Autodesk Fusion 360 part; units mm, degrees
note: some values were not read from the file. Set by a fixed rule: which sketch regions a step uses.
(part 12 of 15)
  line L9703 (42.4168, -64.2747) -> (42.4728, -64.098)
  line L9704 (145.736, -64.6246) -> (145.454, -64.6312)
  line L9705 (143.987, -63.884) -> (143.827, -63.6515)
  line L9706 (184.335, -62.7681) -> (184.478, -62.8863)
  line L9707 (145.579, -60.6337) -> (145.861, -60.6581)
  line L9708 (147.166, -63.809) -> (146.984, -64.0253)
  line L9709 (147.544, -62.759) -> (147.506, -63.039)
  line L9710 (147.43, -63.3109) -> (147.316, -63.5693)
  line L9711 (146.015, -64.5782) -> (145.736, -64.6246)
  line L9712 (145.173, -64.598) -> (144.9, -64.5256)
  line L9713 (147.528, -62.3517) -> (147.548, -62.6335)
  line L9714 (146.4, -60.8238) -> (146.646, -60.9619)
  line L9715 (184.753, -63.5822) -> (184.73, -63.7661)
  line L9716 (143.752, -61.7536) -> (143.894, -61.5093)
  line L9717 (188.432, -64.6381) -> (188.159, -64.5657)
  line L9718 (143.578, -62.2896) -> (143.646, -62.0154)
  line L9719 (144.503, -60.9282) -> (144.754, -60.798)
  line L9720 (144.273, -61.0924) -> (144.503, -60.9282)
  line L9721 (184.172, -62.6799) -> (184.335, -62.7681)
  line L9722 (184.478, -62.8863) -> (184.595, -63.0299)
  line L9723 (145.02, -60.7044) -> (145.297, -60.6492)
  line L9724 (144.069, -61.2874) -> (144.273, -61.0924)
  line L9725 (146.984, -64.0253) -> (146.774, -64.2138)
  line L9726 (189.543, -64.5331) -> (189.273, -64.6183)
  line L9727 (145.861, -60.6581) -> (146.136, -60.7219)
  line L9728 (190.807, -62.6735) -> (190.803, -62.7991)
  line L9729 (188.279, -60.7444) -> (188.556, -60.6893)
  line L9730 (184.595, -63.0299) -> (184.682, -63.1936)
  line L9731 (144.9, -64.5256) -> (144.64, -64.4155)
  line L9732 (147.069, -61.3346) -> (147.237, -61.5618)
  line L9733 (146.646, -60.9619) -> (146.871, -61.1332)
  line L9734 (146.871, -61.1332) -> (147.069, -61.3346)
  line L9735 (187.01, -61.7937) -> (187.152, -61.5494)
  line L9736 (184.682, -63.1936) -> (184.736, -63.3711)
  line L9737 (184.73, -63.7661) -> (184.672, -63.9421)
  line L9738 (186.904, -62.0555) -> (187.01, -61.7937)
  line L9739 (184.672, -63.9421) -> (184.58, -64.1033)
  line L9740 (147.371, -61.8104) -> (147.469, -62.0755)
  line L9741 (187.532, -61.1325) -> (187.762, -60.9683)
  line L9742 (188.159, -64.5657) -> (187.899, -64.4555)
  line L9743 (147.506, -63.039) -> (147.43, -63.3109)
  line L9744 (147.237, -61.5618) -> (147.371, -61.8104)
  line L9745 (147.316, -63.5693) -> (147.166, -63.809)
  line L9746 (146.539, -64.3707) -> (146.284, -64.493)
  line L9747 (190.032, -64.2538) -> (189.797, -64.4108)
  line L9748 (190.495, -61.6019) -> (190.629, -61.8505)
  line L9749 (188.012, -60.838) -> (188.279, -60.7444)
  line L9750 (187.327, -61.3275) -> (187.532, -61.1325)
  line L9751 (189.273, -64.6183) -> (188.995, -64.6647)
  line L9752 (188.556, -60.6893) -> (188.838, -60.6738)
  line L9753 (146.136, -60.7219) -> (146.4, -60.8238)
  line L9754 (188.838, -60.6738) -> (189.119, -60.6982)
  line L9755 (146.284, -64.493) -> (146.015, -64.5782)
  line L9756 (147.548, -62.6335) -> (147.544, -62.759)
  line L9757 (145.454, -64.6312) -> (145.173, -64.598)
  line L9758 (183.995, -62.6251) -> (184.172, -62.6799)
  line L9759 (143.549, -62.5706) -> (143.578, -62.2896)
  line L9760 (144.754, -60.798) -> (145.02, -60.7044)
  line L9761 (143.646, -62.0154) -> (143.752, -61.7536)
  line L9762 (187.762, -60.9683) -> (188.012, -60.838)
  line L9763 (147.469, -62.0755) -> (147.528, -62.3517)
  line L9764 (189.797, -64.4108) -> (189.543, -64.5331)
  line L9765 (145.297, -60.6492) -> (145.579, -60.6337)
  line L9766 (187.152, -61.5494) -> (187.327, -61.3275)
  line L9767 (146.774, -64.2138) -> (146.539, -64.3707)
  line L9768 (182.869, -63.7272) -> (182.854, -63.5424)
  line L9769 (306.287, -60.7875) -> (306.455, -61.0148)
  line L9770 (182.874, -63.3581) -> (182.931, -63.1814)
  line L9771 (151.5, -63.5421) -> (151.477, -63.7261)
  line L9772 (151.342, -62.9899) -> (151.429, -63.1536)
  line L9773 (183.262, -64.3358) -> (183.12, -64.2156)
  line L9774 (182.92, -63.9054) -> (182.869, -63.7272)
  line L9775 (150.373, -62.5824) -> (150.557, -62.5656)
  line L9776 (151.327, -64.0632) -> (151.206, -64.2036)
  line L9777 (149.678, -63.1414) -> (149.767, -62.9789)
  line L9778 (183.81, -62.6057) -> (183.995, -62.6251)
  line L9779 (151.429, -63.1536) -> (151.483, -63.3311)
  line L9780 (150.195, -62.6348) -> (150.373, -62.5824)
  line L9781 (149.767, -62.9789) -> (149.886, -62.8368)
  line L9782 (183.969, -64.4912) -> (183.784, -64.5055)
  line L9783 (149.616, -63.6871) -> (149.601, -63.5023)
  line L9784 (183.448, -62.6748) -> (183.626, -62.6225)
  line L9785 (184.736, -63.3711) -> (184.754, -63.5557)
  line L9786 (184.754, -63.5557) -> (184.753, -63.5822)
  line L9787 (144.179, -64.0914) -> (143.987, -63.884)
  line L9788 (183.02, -63.0189) -> (183.139, -62.8769)
  line L9789 (150.919, -62.6398) -> (151.082, -62.728)
  line L9790 (151.419, -63.902) -> (151.327, -64.0632)
  line L9791 (305.079, -60.111) -> (305.354, -60.1748)
  line L9792 (184.313, -64.3578) -> (184.147, -64.4414)
  line L9793 (150.009, -64.2957) -> (149.867, -64.1755)
  line L9794 (149.886, -62.8368) -> (150.031, -62.7207)
  line L9795 (150.17, -64.3861) -> (150.009, -64.2957)
  line L9796 (151.483, -63.3311) -> (151.501, -63.5156)
  line L9797 (183.423, -64.4262) -> (183.262, -64.3358)
  line L9798 (143.56, -62.8529) -> (143.549, -62.5706)
  line L9799 (143.894, -61.5093) -> (144.069, -61.2874)
  line L9800 (183.284, -62.7607) -> (183.448, -62.6748)
  line L9801 (184.147, -64.4414) -> (183.969, -64.4912)
  line L9802 (184.58, -64.1033) -> (184.459, -64.2436)
  line L9803 (306.687, -61.5284) -> (306.746, -61.8046)
  line L9804 (143.7, -63.3988) -> (143.611, -63.1308)
  line L9805 (149.752, -64.0302) -> (149.668, -63.8653)
  line L9806 (306.589, -61.2634) -> (306.687, -61.5284)
  line L9807 (183.626, -62.6225) -> (183.81, -62.6057)
  line L9808 (151.206, -64.2036) -> (151.06, -64.3177)
  line L9809 (149.668, -63.8653) -> (149.616, -63.6871)
  line L9810 (144.398, -64.2698) -> (144.179, -64.0914)
  line L9811 (143.827, -63.6515) -> (143.7, -63.3988)
  line L9812 (183.6, -64.4835) -> (183.423, -64.4262)
  line L9813 (151.225, -62.8462) -> (151.342, -62.9899)
  line L9814 (151.501, -63.5156) -> (151.5, -63.5421)
  line L9815 (182.854, -63.5424) -> (182.874, -63.3581)
  line L9816 (183.139, -62.8769) -> (183.284, -62.7607)
  line L9817 (182.931, -63.1814) -> (183.02, -63.0189)
  line L9818 (183.784, -64.5055) -> (183.6, -64.4835)
  line L9819 (149.622, -63.3181) -> (149.678, -63.1414)
  line L9820 (305.618, -60.2768) -> (305.864, -60.4148)
  line L9821 (150.031, -62.7207) -> (150.195, -62.6348)
  line L9822 (151.082, -62.728) -> (151.225, -62.8462)
  line L9823 (151.06, -64.3177) -> (150.894, -64.4013)
  line L9824 (151.477, -63.7261) -> (151.419, -63.902)
  line L9825 (183.12, -64.2156) -> (183.005, -64.0703)
  line L9826 (150.716, -64.4512) -> (150.531, -64.4654)
  line L9827 (150.742, -62.585) -> (150.919, -62.6398)
  line L9828 (144.64, -64.4155) -> (144.398, -64.2698)
  line L9829 (143.611, -63.1308) -> (143.56, -62.8529)
  line L9830 (184.459, -64.2436) -> (184.313, -64.3578)
  line L9831 (183.005, -64.0703) -> (182.92, -63.9054)
  line L9832 (306.202, -63.4782) -> (305.992, -63.6667)
  line L9833 (303.858, -63.8684) -> (303.616, -63.7227)
  line L9834 (302.864, -61.4684) -> (302.97, -61.2065)
  line L9835 (306.384, -63.262) -> (306.202, -63.4782)
  line L9836 (305.233, -64.0312) -> (304.954, -64.0775)
  line L9837 (302.97, -61.2065) -> (303.112, -60.9622)
  line L9838 (306.089, -60.5862) -> (306.287, -60.7875)
  line L9839 (302.767, -62.0236) -> (302.796, -61.7426)
  line L9840 (303.491, -60.5454) -> (303.721, -60.3811)
  line L9841 (303.287, -60.7404) -> (303.491, -60.5454)
  line L9842 (303.397, -63.5444) -> (303.205, -63.3369)
  line L9843 (306.766, -62.0864) -> (306.762, -62.212)
  line L9844 (31.5843, -62.1719) -> (31.5467, -62.4519)
  line L9845 (30.6863, -60.3747) -> (30.9109, -60.5461)
  line L9846 (306.648, -62.7639) -> (306.534, -63.0223)
  line L9847 (303.972, -60.2509) -> (304.238, -60.1573)
  line L9848 (31.2769, -60.9747) -> (31.4111, -61.2233)
  line L9849 (302.829, -62.5838) -> (302.778, -62.3059)
  line L9850 (303.721, -60.3811) -> (303.972, -60.2509)
  line L9851 (304.672, -64.0842) -> (304.391, -64.051)
  line L9852 (31.1091, -60.7475) -> (31.2769, -60.9747)
  line L9853 (30.0552, -63.9911) -> (29.7765, -64.0375)
  line L9854 (29.494, -64.0441) -> (29.2135, -64.0109)
  line L9855 (28.4383, -63.6826) -> (28.2192, -63.5043)
  line L9856 (303.616, -63.7227) -> (303.397, -63.5444)
  line L9857 (305.354, -60.1748) -> (305.618, -60.2768)
  line L9858 (29.2135, -64.0109) -> (28.9404, -63.9385)
  line L9859 (30.1763, -60.1348) -> (30.4398, -60.2367)
  line L9860 (302.918, -62.8518) -> (302.829, -62.5838)
  line L9861 (30.8141, -63.6267) -> (30.5792, -63.7836)
  line L9862 (306.725, -62.492) -> (306.648, -62.7639)
  line L9863 (305.992, -63.6667) -> (305.757, -63.8237)
  line L9864 (303.205, -63.3369) -> (303.045, -63.1045)
  line L9865 (304.118, -63.9786) -> (303.858, -63.8684)
  line L9866 (30.5792, -63.7836) -> (30.3245, -63.9059)
  line L9867 (31.3558, -62.9822) -> (31.2063, -63.2219)
  line L9868 (305.502, -63.946) -> (305.233, -64.0312)
  line L9869 (28.6803, -63.8284) -> (28.4383, -63.6826)
  line L9870 (31.5467, -62.4519) -> (31.47, -62.7238)
  line L9871 (306.455, -61.0148) -> (306.589, -61.2634)
  line L9872 (302.796, -61.7426) -> (302.864, -61.4684)
  line L9873 (306.534, -63.0223) -> (306.384, -63.262)
  line L9874 (303.045, -63.1045) -> (302.918, -62.8518)
  line L9875 (303.112, -60.9622) -> (303.287, -60.7404)
  line L9876 (304.391, -64.051) -> (304.118, -63.9786)
  line L9877 (304.954, -64.0775) -> (304.672, -64.0842)
  line L9878 (306.762, -62.212) -> (306.725, -62.492)
  line L9879 (302.778, -62.3059) -> (302.767, -62.0236)
  line L9880 (305.757, -63.8237) -> (305.502, -63.946)
  line L9881 (29.7765, -64.0375) -> (29.494, -64.0441)
  line L9882 (31.5883, -62.0463) -> (31.5843, -62.1719)
  line L9883 (28.2192, -63.5043) -> (28.0274, -63.2968)
  line L9884 (28.9404, -63.9385) -> (28.6803, -63.8284)
  line L9885 (150.531, -64.4654) -> (150.347, -64.4434)
  line L9886 (306.746, -61.8046) -> (306.766, -62.0864)
  line L9887 (30.3245, -63.9059) -> (30.0552, -63.9911)
  line L9888 (304.516, -60.1022) -> (304.798, -60.0867)
  line L9889 (29.9011, -60.071) -> (30.1763, -60.1348)
  line L9890 (305.864, -60.4148) -> (306.089, -60.5862)
  line L9891 (149.867, -64.1755) -> (149.752, -64.0302)
  line L9892 (150.347, -64.4434) -> (150.17, -64.3861)
  line L9893 (150.894, -64.4013) -> (150.716, -64.4512)
  line L9894 (149.601, -63.5023) -> (149.622, -63.3181)
  line L9895 (150.557, -62.5656) -> (150.742, -62.585)
  line L9896 (35.2652, -62.2591) -> (35.3824, -62.4028)
  line L9897 (300.107, -63.8543) -> (299.928, -63.9041)
  line L9898 (299.221, -63.7486) -> (299.08, -63.6285)
  line L9899 (31.2063, -63.2219) -> (31.0245, -63.4382)
  line L9900 (300.713, -62.9685) -> (300.713, -62.9951)
  line L9901 (300.295, -62.181) -> (300.438, -62.2991)
  line L9902 (299.744, -63.9183) -> (299.559, -63.8964)
  line L9903 (35.5175, -63.139) -> (35.459, -63.3149)
  line L9904 (298.834, -62.771) -> (298.89, -62.5943)
  line L9905 (30.4398, -60.2367) -> (30.6863, -60.3747)
  line L9906 (31.5683, -61.7645) -> (31.5883, -62.0463)
  line L9907 (34.7821, -61.9979) -> (34.9592, -62.0527)
  line L9908 (35.3824, -62.4028) -> (35.4694, -62.5665)
  line L9909 (299.954, -62.038) -> (300.132, -62.0928)
  line L9910 (299.383, -63.8391) -> (299.221, -63.7486)
  line L9911 (35.459, -63.3149) -> (35.3674, -63.4761)
  line L9912 (27.6511, -62.5437) -> (27.6003, -62.2658)
  line L9913 (300.419, -63.6565) -> (300.272, -63.7707)
  line L9914 (27.7405, -62.8117) -> (27.6511, -62.5437)
  line L9915 (31.47, -62.7238) -> (31.3558, -62.9822)
  line L9916 (31.4111, -61.2233) -> (31.5088, -61.4884)
  line L9917 (28.794, -60.2108) -> (29.0605, -60.1172)
  line L9918 (27.7922, -61.1665) -> (27.9341, -60.9222)
  line L9919 (28.109, -60.7003) -> (28.3134, -60.5053)
  line L9920 (304.798, -60.0867) -> (305.079, -60.111)
  line L9921 (300.642, -62.6065) -> (300.695, -62.784)
  line L9922 (28.0274, -63.2968) -> (27.8668, -63.0644)
  line L9923 (300.631, -63.3549) -> (300.54, -63.5162)
  line L9924 (300.555, -62.4428) -> (300.642, -62.6065)
  line L9925 (300.272, -63.7707) -> (300.107, -63.8543)
  line L9926 (28.5433, -60.3411) -> (28.794, -60.2108)
  line L9927 (31.0245, -63.4382) -> (30.8141, -63.6267)
  line L9928 (27.618, -61.7025) -> (27.6861, -61.4283)
  line L9929 (298.98, -62.4318) -> (299.099, -62.2898)
  line L9930 (29.3376, -60.0621) -> (29.6197, -60.0466)
  line L9931 (35.523, -62.744) -> (35.5411, -62.9285)
  line L9932 (298.88, -63.3183) -> (298.829, -63.14)
  line L9933 (27.5892, -61.9835) -> (27.618, -61.7025)
  line L9934 (35.5407, -62.955) -> (35.5175, -63.139)
  line L9935 (29.6197, -60.0466) -> (29.9011, -60.071)
  line L9936 (31.5088, -61.4884) -> (31.5683, -61.7645)
  line L9937 (300.54, -63.5162) -> (300.419, -63.6565)
  line L9938 (300.713, -62.9951) -> (300.69, -63.179)
  line L9939 (27.9341, -60.9222) -> (28.109, -60.7003)
  line L9940 (300.695, -62.784) -> (300.713, -62.9685)
  line L9941 (35.4694, -62.5665) -> (35.523, -62.744)
  line L9942 (299.08, -63.6285) -> (298.965, -63.4832)
  line L9943 (30.9109, -60.5461) -> (31.1091, -60.7475)
  line L9944 (27.6003, -62.2658) -> (27.5892, -61.9835)
  line L9945 (304.238, -60.1573) -> (304.516, -60.1022)
  line L9946 (300.69, -63.179) -> (300.631, -63.3549)
  line L9947 (300.438, -62.2991) -> (300.555, -62.4428)
  line L9948 (27.6861, -61.4283) -> (27.7922, -61.1665)
  line L9949 (298.829, -63.14) -> (298.814, -62.9553)
  line L9950 (35.3674, -63.4761) -> (35.2462, -63.6164)
  line L9951 (35.2462, -63.6164) -> (35.1001, -63.7306)
  line L9952 (298.814, -62.9553) -> (298.834, -62.771)
  line L9953 (35.5411, -62.9285) -> (35.5407, -62.955)
  line L9954 (298.89, -62.5943) -> (298.98, -62.4318)
  line L9955 (28.3134, -60.5053) -> (28.5433, -60.3411)
  line L9956 (27.8668, -63.0644) -> (27.7405, -62.8117)
  line L9957 (300.132, -62.0928) -> (300.295, -62.181)
  line L9958 (29.0605, -60.1172) -> (29.3376, -60.0621)
  line L9959 (299.77, -62.0186) -> (299.954, -62.038)
  line L9960 (34.2108, -63.799) -> (34.0489, -63.7086)
  line L9961 (34.5712, -63.8783) -> (34.3871, -63.8563)
  line L9962 (157.911, -61.7807) -> (158.031, -61.6546)
  line L9963 (33.6567, -63.1) -> (33.6412, -62.9152)
  line L9964 (157.963, -62.7415) -> (157.861, -62.6016)
  line L9965 (298.965, -63.4832) -> (298.88, -63.3183)
  line L9966 (299.585, -62.0354) -> (299.77, -62.0186)
  line L9967 (159.605, -61.4858) -> (159.773, -61.527)
  line L9968 (299.408, -62.0877) -> (299.585, -62.0354)
  line L9969 (159.928, -61.606) -> (160.061, -61.7185)
  line L9970 (160.163, -61.8584) -> (160.231, -62.0182)
  line L9971 (158.031, -61.6546) -> (158.176, -61.5594)
  line L9972 (176.088, -62.9006) -> (175.925, -62.9599)
  line L9973 (157.824, -61.9309) -> (157.911, -61.7807)
  line L9974 (34.0709, -62.1336) -> (34.2352, -62.0477)
  line L9975 (176.233, -62.8054) -> (176.088, -62.9006)
  line L9976 (175.752, -62.98) -> (174.752, -62.98)
  line L9977 (33.7078, -63.2782) -> (33.6567, -63.1)
  line L9978 (176.49, -62.3628) -> (176.44, -62.5291)
  line L9979 (34.5977, -61.9785) -> (34.7821, -61.9979)
  line L9980 (33.7179, -62.5542) -> (33.8072, -62.3918)
  line L9981 (35.1001, -63.7306) -> (34.9346, -63.8142)
  line L9982 (176.471, -62.0182) -> (176.501, -62.1894)
  line L9983 (159.512, -62.98) -> (158.512, -62.98)
  line L9984 (160.261, -62.1894) -> (160.25, -62.3628)
  line L9985 (159.685, -62.9599) -> (159.512, -62.98)
  line L9986 (158.096, -62.854) -> (157.963, -62.7415)
  line L9987 (176.013, -61.527) -> (176.168, -61.606)
  line L9988 (175.925, -62.9599) -> (175.752, -62.98)
  line L9989 (33.6412, -62.9152) -> (33.6618, -62.731)
  line L9990 (33.7925, -63.4431) -> (33.7078, -63.2782)
  line L9991 (34.7561, -63.864) -> (34.5712, -63.8783)
  line L9992 (34.4131, -61.9953) -> (34.5977, -61.9785)
  line L9993 (33.9264, -62.2497) -> (34.0709, -62.1336)
  line L9994 (33.8072, -62.3918) -> (33.9264, -62.2497)
  line L9995 (157.793, -62.4418) -> (157.763, -62.2706)
  line L9996 (176.501, -62.1894) -> (176.49, -62.3628)
  line L9997 (299.099, -62.2898) -> (299.243, -62.1736)
  line L9998 (299.928, -63.9041) -> (299.744, -63.9183)
  line L9999 (34.2352, -62.0477) -> (34.4131, -61.9953)
  line L10000 (159.773, -61.527) -> (159.928, -61.606)
  line L10001 (176.353, -62.6793) -> (176.233, -62.8054)
  line L10002 (157.763, -62.2706) -> (157.774, -62.0972)
  line L10003 (158.176, -61.5594) -> (158.339, -61.5001)
  line L10004 (158.251, -62.933) -> (158.096, -62.854)
  line L10005 (157.861, -62.6016) -> (157.793, -62.4418)
  line L10006 (299.243, -62.1736) -> (299.408, -62.0877)
  line L10007 (160.25, -62.3628) -> (160.2, -62.5291)
  line L10008 (158.339, -61.5001) -> (158.512, -61.48)
  line L10009 (34.0489, -63.7086) -> (33.9077, -63.5884)
  line L10010 (160.061, -61.7185) -> (160.163, -61.8584)
  line L10011 (158.419, -62.9742) -> (158.251, -62.933)
  line L10012 (33.6618, -62.731) -> (33.7179, -62.5542)
  line L10013 (299.559, -63.8964) -> (299.383, -63.8391)
  line L10014 (35.1223, -62.1409) -> (35.2652, -62.2591)
  line L10015 (34.3871, -63.8563) -> (34.2108, -63.799)
  line L10016 (160.231, -62.0182) -> (160.261, -62.1894)
  line L10017 (160.2, -62.5291) -> (160.113, -62.6793)
  line L10018 (159.993, -62.8054) -> (159.848, -62.9006)
  line L10019 (34.9346, -63.8142) -> (34.7561, -63.864)
  line L10020 (34.9592, -62.0527) -> (35.1223, -62.1409)
  line L10021 (33.9077, -63.5884) -> (33.7925, -63.4431)
  line L10022 (160.113, -62.6793) -> (159.993, -62.8054)
  line L10023 (159.848, -62.9006) -> (159.685, -62.9599)
  line L10024 (174.579, -61.5001) -> (174.752, -61.48)
  line L10025 (176.44, -62.5291) -> (176.353, -62.6793)
  line L10026 (194.736, -62.0019) -> (194.677, -62.1778)
  line L10027 (174.491, -62.933) -> (174.336, -62.854)
  line L10028 (174.752, -62.98) -> (174.659, -62.9742)
  line L10029 (194.601, -61.2657) -> (194.688, -61.4294)
  line L10030 (174.271, -61.6546) -> (174.416, -61.5594)
  line L10031 (141.413, -62.1377) -> (141.321, -62.2989)
  line L10032 (192.88, -61.5939) -> (192.936, -61.4172)
  line L10033 (174.151, -61.7807) -> (174.271, -61.6546)
  line L10034 (174.101, -62.6016) -> (174.033, -62.4418)
  line L10035 (194.759, -61.8179) -> (194.736, -62.0019)
  line L10036 (192.875, -61.9629) -> (192.859, -61.7781)
  line L10037 (193.789, -62.7412) -> (193.605, -62.7192)
  line L10038 (193.011, -62.306) -> (192.926, -62.1411)
  line L10039 (141.477, -61.5668) -> (141.495, -61.7513)
  line L10040 (158.512, -62.98) -> (158.419, -62.9742)
  line L10041 (158.512, -61.48) -> (159.512, -61.48)
  line L10042 (194.153, -62.6771) -> (193.974, -62.727)
  line L10043 (194.177, -60.9156) -> (194.341, -61.0038)
  line L10044 (174.033, -62.4418) -> (174.003, -62.2706)
  line L10045 (194.341, -61.0038) -> (194.483, -61.122)
  line L10046 (194.677, -62.1778) -> (194.586, -62.339)
  line L10047 (193.145, -61.1126) -> (193.289, -60.9965)
  line L10048 (176.168, -61.606) -> (176.301, -61.7185)
  line L10049 (176.301, -61.7185) -> (176.403, -61.8584)
  line L10050 (174.752, -61.48) -> (175.752, -61.48)
  line L10051 (193.816, -60.8414) -> (194, -60.8608)
  line L10052 (194.318, -62.5935) -> (194.153, -62.6771)
  line L10053 (157.774, -62.0972) -> (157.824, -61.9309)
  line L10054 (141.076, -60.9637) -> (141.219, -61.0819)
  line L10055 (194.483, -61.122) -> (194.601, -61.2657)
  line L10056 (174.003, -62.2706) -> (174.014, -62.0972)
  line L10057 (141.054, -62.5534) -> (140.889, -62.637)
  line L10058 (194.464, -62.4794) -> (194.318, -62.5935)
  line L10059 (192.859, -61.7781) -> (192.88, -61.5939)
  line L10060 (140.736, -60.8207) -> (140.913, -60.8756)
  line L10061 (193.267, -62.5715) -> (193.126, -62.4513)
  line L10062 (141.321, -62.2989) -> (141.2, -62.4393)
  line L10063 (175.845, -61.4858) -> (176.013, -61.527)
  line L10064 (174.336, -62.854) -> (174.203, -62.7415)
  line L10065 (194.586, -62.339) -> (194.464, -62.4794)
  line L10066 (159.512, -61.48) -> (159.605, -61.4858)
  line L10067 (193.429, -62.6619) -> (193.267, -62.5715)
  line L10068 (174.416, -61.5594) -> (174.579, -61.5001)
  line L10069 (140.913, -60.8756) -> (141.076, -60.9637)
  line L10070 (174.203, -62.7415) -> (174.101, -62.6016)
  line L10071 (175.752, -61.48) -> (175.845, -61.4858)
  line L10072 (174.659, -62.9742) -> (174.491, -62.933)
  line L10073 (193.289, -60.9965) -> (193.453, -60.9106)
  line L10074 (192.936, -61.4172) -> (193.025, -61.2547)
  line L10075 (193.631, -60.8582) -> (193.816, -60.8414)
  line L10076 (193.126, -62.4513) -> (193.011, -62.306)
  line L10077 (193.025, -61.2547) -> (193.145, -61.1126)
  line L10078 (141.2, -62.4393) -> (141.054, -62.5534)
  line L10079 (140.889, -62.637) -> (140.71, -62.6869)
  line L10080 (194.688, -61.4294) -> (194.741, -61.6069)
  line L10081 (193.974, -62.727) -> (193.789, -62.7412)
  line L10082 (174.014, -62.0972) -> (174.064, -61.9309)
  line L10083 (176.403, -61.8584) -> (176.471, -62.0182)
  line L10084 (194.759, -61.7914) -> (194.759, -61.8179)
  line L10085 (174.064, -61.9309) -> (174.151, -61.7807)
  line L10086 (194.741, -61.6069) -> (194.759, -61.7914)
  line L10087 (194, -60.8608) -> (194.177, -60.9156)
  line L10088 (140.552, -60.8014) -> (140.736, -60.8207)
  line L10089 (141.423, -61.3893) -> (141.477, -61.5668)
  line L10090 (139.761, -61.2146) -> (139.88, -61.0726)
  line L10091 (140.025, -60.9564) -> (140.189, -60.8705)
  line L10092 (310.545, -61.7519) -> (310.424, -61.8922)
  line L10093 (140.525, -62.7011) -> (140.341, -62.6792)
  line L10094 (310.424, -61.8922) -> (310.278, -62.0064)
  line L10095 (310.278, -62.0064) -> (310.113, -62.09)
  line L10096 (310.719, -61.2043) -> (310.719, -61.2308)
  line L10097 (310.719, -61.2308) -> (310.695, -61.4148)
  line L10098 (140.189, -60.8705) -> (140.367, -60.8182)
  line L10099 (310.113, -62.09) -> (309.934, -62.1398)
  line L10100 (310.701, -61.0198) -> (310.719, -61.2043)
  line L10101 (140.003, -62.5314) -> (139.862, -62.4113)
  line L10102 (310.637, -61.5907) -> (310.545, -61.7519)
  line L10103 (24.7765, -60.2336) -> (24.9536, -60.2884)
  line L10104 (141.472, -61.9618) -> (141.413, -62.1377)
  line L10105 (310.3, -60.4167) -> (310.443, -60.5349)
  line L10106 (308.985, -60.6676) -> (309.104, -60.5255)
  line L10107 (25.3767, -60.6385) -> (25.4638, -60.8022)
  line L10108 (25.5354, -61.1642) -> (25.5351, -61.1907)
  line L10109 (141.219, -61.0819) -> (141.336, -61.2256)
  line L10110 (139.747, -62.266) -> (139.662, -62.1011)
  line L10111 (25.1167, -60.3766) -> (25.2595, -60.4948)
  line L10112 (193.605, -62.7192) -> (193.429, -62.6619)
  line L10113 (140.165, -62.6219) -> (140.003, -62.5314)
  line L10114 (309.934, -62.1398) -> (309.749, -62.1541)
  line L10115 (25.3617, -61.7118) -> (25.2406, -61.8522)
  line L10116 (139.88, -61.0726) -> (140.025, -60.9564)
  line L10117 (140.71, -62.6869) -> (140.525, -62.7011)
  line L10118 (310.695, -61.4148) -> (310.637, -61.5907)
  line L10119 (192.926, -62.1411) -> (192.875, -61.9629)
  line L10120 (309.591, -60.2711) -> (309.776, -60.2543)
  line L10121 (25.4638, -60.8022) -> (25.5173, -60.9797)
  line L10122 (25.5118, -61.3747) -> (25.4533, -61.5506)
  line L10123 (25.4533, -61.5506) -> (25.3617, -61.7118)
  line L10124 (308.896, -60.83) -> (308.985, -60.6676)
  line L10125 (310.137, -60.3285) -> (310.3, -60.4167)
  line L10126 (309.96, -60.2737) -> (310.137, -60.3285)
  line L10127 (139.616, -61.5538) -> (139.672, -61.3771)
  line L10128 (308.819, -61.191) -> (308.84, -61.0068)
  line L10129 (309.776, -60.2543) -> (309.96, -60.2737)
  line L10130 (309.249, -60.4094) -> (309.413, -60.3235)
  line L10131 (25.2406, -61.8522) -> (25.0945, -61.9663)
  line L10132 (310.56, -60.6786) -> (310.647, -60.8423)
  line L10133 (139.672, -61.3771) -> (139.761, -61.2146)
  line L10134 (193.453, -60.9106) -> (193.631, -60.8582)
  line L10135 (141.495, -61.7513) -> (141.495, -61.7779)
  line L10136 (140.367, -60.8182) -> (140.552, -60.8014)
  line L10137 (25.5173, -60.9797) -> (25.5354, -61.1642)
  line L10138 (308.971, -61.7189) -> (308.886, -61.554)
  line L10139 (25.0945, -61.9663) -> (24.929, -62.0499)
  line L10140 (308.886, -61.554) -> (308.835, -61.3758)
  line L10141 (139.862, -62.4113) -> (139.747, -62.266)
  line L10142 (25.2595, -60.4948) -> (25.3767, -60.6385)
  line L10143 (309.086, -61.8642) -> (308.971, -61.7189)
  line L10144 (140.341, -62.6792) -> (140.165, -62.6219)
  line L10145 (310.443, -60.5349) -> (310.56, -60.6786)
  line L10146 (139.662, -62.1011) -> (139.611, -61.9228)
  line L10147 (141.336, -61.2256) -> (141.423, -61.3893)
  line L10148 (139.611, -61.9228) -> (139.595, -61.7381)
  line L10149 (310.647, -60.8423) -> (310.701, -61.0198)
  line L10150 (139.595, -61.7381) -> (139.616, -61.5538)
  line L10151 (141.495, -61.7779) -> (141.472, -61.9618)
  line L10152 (4.2421, -61.7096) -> (3.9635, -61.756)
  line L10153 (3.9635, -61.756) -> (3.681, -61.7627)
  line L10154 (2.5004, -58.2239) -> (2.7302, -58.0596)
  line L10155 (23.9208, -60.4855) -> (24.0653, -60.3693)
  line L10156 (1.8381, -60.2623) -> (1.7873, -59.9844)
  line L10157 (23.6355, -61.151) -> (23.6562, -60.9667)
  line L10158 (2.9809, -57.9294) -> (3.2475, -57.8358)
  line L10159 (24.2051, -62.0348) -> (24.0433, -61.9443)
  line L10160 (3.2475, -57.8358) -> (3.5246, -57.7807)
  line L10161 (23.9021, -61.8241) -> (23.7869, -61.6788)
  line L10162 (23.651, -61.3357) -> (23.6355, -61.151)
  line L10163 (1.805, -59.421) -> (1.8731, -59.1469)
  line L10164 (5.3933, -60.9405) -> (5.2115, -61.1567)
  line L10165 (24.929, -62.0499) -> (24.7504, -62.0998)
  line L10166 (24.5921, -60.2142) -> (24.7765, -60.2336)
  line L10167 (3.5246, -57.7807) -> (3.8067, -57.7652)
  line L10168 (2.296, -58.4189) -> (2.5004, -58.2239)
  line L10169 (309.389, -62.0748) -> (309.227, -61.9844)
  line L10170 (5.7713, -59.8905) -> (5.7337, -60.1705)
  line L10171 (5.598, -58.9419) -> (5.6958, -59.2069)
  line L10172 (24.0653, -60.3693) -> (24.2296, -60.2834)
  line L10173 (5.4639, -58.6933) -> (5.598, -58.9419)
  line L10174 (23.7869, -61.6788) -> (23.7021, -61.5139)
  line L10175 (1.7762, -59.7021) -> (1.805, -59.421)
  line L10176 (24.2296, -60.2834) -> (24.4074, -60.231)
  line L10177 (308.84, -61.0068) -> (308.896, -60.83)
  line L10178 (24.4074, -60.231) -> (24.5921, -60.2142)
  line L10179 (23.6562, -60.9667) -> (23.7123, -60.79)
  line L10180 (3.681, -61.7627) -> (3.4005, -61.7295)
  line L10181 (1.8731, -59.1469) -> (1.9792, -58.885)
  line L10182 (2.1211, -58.6407) -> (2.296, -58.4189)
  line L10183 (5.7752, -59.7649) -> (5.7713, -59.8905)
  line L10184 (23.8016, -60.6275) -> (23.9208, -60.4855)
  line L10185 (3.4005, -61.7295) -> (3.1274, -61.6571)
  line L10186 (24.3814, -62.0921) -> (24.2051, -62.0348)
  line L10187 (2.7302, -58.0596) -> (2.9809, -57.9294)
  line L10188 (5.0011, -61.3452) -> (4.7661, -61.5022)
  line L10189 (24.7504, -62.0998) -> (24.5655, -62.114)
  line L10190 (309.749, -62.1541) -> (309.565, -62.1321)
  line L10191 (24.5655, -62.114) -> (24.3814, -62.0921)
  line L10192 (5.2961, -58.466) -> (5.4639, -58.6933)
  line L10193 (4.5115, -61.6245) -> (4.2421, -61.7096)
  line L10194 (1.7873, -59.9844) -> (1.7762, -59.7021)
  line L10195 (5.0979, -58.2647) -> (5.2961, -58.466)
  line L10196 (5.7553, -59.4831) -> (5.7752, -59.7649)
  line L10197 (2.2144, -61.0154) -> (2.0537, -60.783)
  line L10198 (1.9275, -60.5303) -> (1.8381, -60.2623)
  line L10199 (4.8733, -58.0933) -> (5.0979, -58.2647)
  line L10200 (5.6958, -59.2069) -> (5.7553, -59.4831)
  line L10201 (23.7021, -61.5139) -> (23.651, -61.3357)
  line L10202 (24.0433, -61.9443) -> (23.9021, -61.8241)
  line L10203 (5.7337, -60.1705) -> (5.657, -60.4424)
  line L10204 (309.227, -61.9844) -> (309.086, -61.8642)
  line L10205 (309.565, -62.1321) -> (309.389, -62.0748)
  line L10206 (24.9536, -60.2884) -> (25.1167, -60.3766)
  line L10207 (309.413, -60.3235) -> (309.591, -60.2711)
  line L10208 (309.104, -60.5255) -> (309.249, -60.4094)
  line L10209 (308.835, -61.3758) -> (308.819, -61.191)
  line L10210 (23.7123, -60.79) -> (23.8016, -60.6275)
  line L10211 (5.657, -60.4424) -> (5.5428, -60.7008)
  line L10212 (4.3633, -57.8533) -> (4.6268, -57.9553)
  line L10213 (4.0881, -57.7895) -> (4.3633, -57.8533)
  line L10214 (25.5351, -61.1907) -> (25.5118, -61.3747)
  line L10215 (4.6268, -57.9553) -> (4.8733, -58.0933)
  line L10216 (9.3093, -59.8595) -> (9.4521, -59.9776)
  line L10217 (4.7661, -61.5022) -> (4.5115, -61.6245)
  line L10218 (7.9942, -60.1103) -> (8.1134, -59.9683)
  line L10219 (9.7281, -60.647) -> (9.7277, -60.6736)
  line L10220 (8.3977, -61.5176) -> (8.2359, -61.4271)
  line L10221 (9.1462, -59.7713) -> (9.3093, -59.8595)
  line L10222 (8.943, -61.5826) -> (8.7582, -61.5968)
  line L10223 (8.5741, -61.5749) -> (8.3977, -61.5176)
  line L10224 (209.526, -59.7711) -> (209.449, -60.043)
  line L10225 (9.4332, -61.335) -> (9.2871, -61.4492)
  line L10226 (208.89, -57.8653) -> (209.088, -58.0666)
  line L10227 (207.192, -61.3301) -> (206.919, -61.2577)
  line L10228 (208.155, -57.4539) -> (208.419, -57.5559)
  line L10229 (5.5428, -60.7008) -> (5.3933, -60.9405)
  line L10230 (206.198, -60.8235) -> (206.006, -60.616)
  line L10231 (206.417, -61.0018) -> (206.198, -60.8235)
  line L10232 (7.8948, -60.9968) -> (7.8437, -60.8185)
  line L10233 (1.9792, -58.885) -> (2.1211, -58.6407)
  line L10234 (7.8437, -60.8185) -> (7.8282, -60.6338)
  line L10235 (206.006, -60.616) -> (205.846, -60.3836)
  line L10236 (9.5543, -61.1947) -> (9.4332, -61.335)
  line L10237 (9.6564, -60.285) -> (9.71, -60.4625)
  line L10238 (207.755, -61.3567) -> (207.473, -61.3633)
  line L10239 (7.9795, -61.1617) -> (7.8948, -60.9968)
  line L10240 (206.659, -61.1475) -> (206.417, -61.0018)
  line L10241 (9.7277, -60.6736) -> (9.7044, -60.8575)
  line L10242 (9.71, -60.4625) -> (9.7281, -60.647)
  line L10243 (208.665, -57.6939) -> (208.89, -57.8653)
  line L10244 (2.0537, -60.783) -> (1.9275, -60.5303)
  line L10245 (7.8282, -60.6338) -> (7.8488, -60.4495)
  line L10246 (9.1216, -61.5327) -> (8.943, -61.5826)
  line L10247 (9.2871, -61.4492) -> (9.1216, -61.5327)
  line L10248 (208.558, -61.1028) -> (208.303, -61.2251)
  line L10249 (209.567, -59.3655) -> (209.563, -59.4911)
  line L10250 (207.473, -61.3633) -> (207.192, -61.3301)
  line L10251 (205.846, -60.3836) -> (205.719, -60.1309)
  line L10252 (8.9691, -59.7164) -> (9.1462, -59.7713)
  line L10253 (9.4521, -59.9776) -> (9.5693, -60.1213)
  line L10254 (8.0947, -61.307) -> (7.9795, -61.1617)
  line L10255 (8.1134, -59.9683) -> (8.2579, -59.8521)
  line L10256 (9.6459, -61.0334) -> (9.5543, -61.1947)
  line L10257 (3.1274, -61.6571) -> (2.8673, -61.5469)
  line L10258 (8.6, -59.7139) -> (8.7847, -59.6971)
  line L10259 (209.088, -58.0666) -> (209.256, -58.2939)
  line L10260 (2.6252, -61.4012) -> (2.4061, -61.2228)
  line L10261 (7.8488, -60.4495) -> (7.9049, -60.2728)
  line L10262 (8.4222, -59.7662) -> (8.6, -59.7139)
  line L10263 (9.5693, -60.1213) -> (9.6564, -60.285)
  line L10264 (8.7582, -61.5968) -> (8.5741, -61.5749)
  line L10265 (208.793, -60.9458) -> (208.558, -61.1028)
  line L10266 (209.547, -59.0837) -> (209.567, -59.3655)
  line L10267 (8.7847, -59.6971) -> (8.9691, -59.7164)
  line L10268 (209.563, -59.4911) -> (209.526, -59.7711)
  line L10269 (7.9049, -60.2728) -> (7.9942, -60.1103)
  line L10270 (206.919, -61.2577) -> (206.659, -61.1475)
  line L10271 (209.39, -58.5425) -> (209.488, -58.8076)
  line L10272 (209.488, -58.8076) -> (209.547, -59.0837)
  line L10273 (3.8067, -57.7652) -> (4.0881, -57.7895)
  line L10274 (5.2115, -61.1567) -> (5.0011, -61.3452)
  line L10275 (9.7044, -60.8575) -> (9.6459, -61.0334)
  line L10276 (2.4061, -61.2228) -> (2.2144, -61.0154)
  line L10277 (8.2579, -59.8521) -> (8.4222, -59.7662)
  line L10278 (2.8673, -61.5469) -> (2.6252, -61.4012)
  line L10279 (8.2359, -61.4271) -> (8.0947, -61.307)
  line L10280 (205.568, -59.3027) -> (205.597, -59.0217)
  line L10281 (205.63, -59.8629) -> (205.579, -59.585)
  line L10282 (128.476, -58.2538) -> (128.61, -58.5024)
  line L10283 (205.913, -58.2414) -> (206.088, -58.0195)
  line L10284 (128.013, -60.9058) -> (127.778, -61.0627)
  line L10285 (128.11, -57.8252) -> (128.308, -58.0266)
  line L10286 (208.419, -57.5559) -> (208.665, -57.6939)
  line L10287 (128.61, -58.5024) -> (128.708, -58.7675)
  line L10288 (128.787, -59.3255) -> (128.783, -59.451)
  line L10289 (127.375, -57.4139) -> (127.639, -57.5158)
  line L10290 (207.039, -57.4364) -> (207.316, -57.3813)
  line L10291 (126.819, -57.3257) -> (127.1, -57.3501)
  line L10292 (124.991, -58.4456) -> (125.133, -58.2013)
  line L10293 (202.932, -59.3719) -> (203.096, -59.4601)
  line L10294 (209.449, -60.043) -> (209.335, -60.3014)
  line L10295 (205.665, -58.7475) -> (205.771, -58.4857)
  line L10296 (128.224, -60.7173) -> (128.013, -60.9058)
  line L10297 (205.719, -60.1309) -> (205.63, -59.8629)
  line L10298 (207.599, -57.3658) -> (207.88, -57.3902)
  line L10299 (207.88, -57.3902) -> (208.155, -57.4539)
  line L10300 (206.292, -57.8245) -> (206.522, -57.6603)
  line L10301 (209.003, -60.7574) -> (208.793, -60.9458)
  line L10302 (128.555, -60.2613) -> (128.405, -60.501)
  line L10303 (205.771, -58.4857) -> (205.913, -58.2414)
  line L10304 (126.413, -61.29) -> (126.14, -61.2176)
  line L10305 (125.227, -60.576) -> (125.066, -60.3436)
  line L10306 (125.742, -57.6202) -> (125.993, -57.49)
  line L10307 (126.537, -57.3412) -> (126.819, -57.3257)
  line L10308 (125.993, -57.49) -> (126.26, -57.3964)
  line L10309 (128.767, -59.0437) -> (128.787, -59.3255)
  line L10310 (128.746, -59.731) -> (128.669, -60.0029)
  line L10311 (126.14, -61.2176) -> (125.879, -61.1075)
  line L10312 (125.308, -57.9794) -> (125.513, -57.7844)
  line L10313 (124.799, -59.5449) -> (124.788, -59.2626)
  line L10314 (125.879, -61.1075) -> (125.637, -60.9618)
  line L10315 (124.85, -59.8228) -> (124.799, -59.5449)
  line L10316 (209.185, -60.5411) -> (209.003, -60.7574)
  line L10317 (127.885, -57.6539) -> (128.11, -57.8252)
  line L10318 (124.885, -58.7074) -> (124.991, -58.4456)
  line L10319 (207.316, -57.3813) -> (207.599, -57.3658)
  line L10320 (203.356, -59.7219) -> (203.443, -59.8856)
  line L10321 (126.26, -57.3964) -> (126.537, -57.3412)
  line L10322 (128.308, -58.0266) -> (128.476, -58.2538)
  line L10323 (128.783, -59.451) -> (128.746, -59.731)
  line L10324 (127.1, -57.3501) -> (127.375, -57.4139)
  line L10325 (206.522, -57.6603) -> (206.773, -57.53)
  line L10326 (209.335, -60.3014) -> (209.185, -60.5411)
  line L10327 (206.773, -57.53) -> (207.039, -57.4364)
  line L10328 (128.405, -60.501) -> (128.224, -60.7173)
  line L10329 (125.513, -57.7844) -> (125.742, -57.6202)
  line L10330 (127.778, -61.0627) -> (127.524, -61.185)
  line L10331 (124.817, -58.9816) -> (124.885, -58.7074)
  line L10332 (208.034, -61.3103) -> (207.755, -61.3567)
  line L10333 (128.669, -60.0029) -> (128.555, -60.2613)
  line L10334 (206.088, -58.0195) -> (206.292, -57.8245)
  line L10335 (126.693, -61.3232) -> (126.413, -61.29)
  line L10336 (203.238, -59.5783) -> (203.356, -59.7219)
  line L10337 (208.303, -61.2251) -> (208.034, -61.3103)
  line L10338 (128.708, -58.7675) -> (128.767, -59.0437)
  line L10339 (205.579, -59.585) -> (205.568, -59.3027)
  line L10340 (205.597, -59.0217) -> (205.665, -58.7475)
  line L10341 (203.096, -59.4601) -> (203.238, -59.5783)
  line L10342 (127.639, -57.5158) -> (127.885, -57.6539)
  line L10343 (209.256, -58.2939) -> (209.39, -58.5425)
  line L10344 (202.044, -59.4527) -> (202.208, -59.3668)
  line L10345 (203.443, -59.8856) -> (203.496, -60.0631)
  line L10346 (125.637, -60.9618) -> (125.418, -60.7834)
  line L10347 (132.669, -59.8456) -> (132.722, -60.0231)
  line L10348 (201.78, -59.7109) -> (201.9, -59.5689)
  line L10349 (202.571, -59.2977) -> (202.755, -59.3171)
  line L10350 (130.861, -60.0101) -> (130.917, -59.8334)
  line L10351 (202.208, -59.3668) -> (202.386, -59.3145)
  line L10352 (131.955, -61.1432) -> (131.77, -61.1574)
  line L10353 (132.464, -59.5382) -> (132.582, -59.6819)
  line L10354 (132.722, -60.0231) -> (132.74, -60.2076)
  line L10355 (131.586, -61.1354) -> (131.41, -61.0781)
  line L10356 (131.612, -59.2744) -> (131.797, -59.2576)
  line L10357 (132.134, -61.0933) -> (131.955, -61.1432)
  line L10358 (131.797, -59.2576) -> (131.981, -59.277)
  line L10359 (131.27, -59.4127) -> (131.434, -59.3268)
  line L10360 (201.9, -59.5689) -> (202.044, -59.4527)
  line L10361 (125.066, -60.3436) -> (124.94, -60.0908)
  line L10362 (203.432, -60.6341) -> (203.341, -60.7953)
  line L10363 (130.84, -60.1943) -> (130.861, -60.0101)
  line L10364 (203.219, -60.9356) -> (203.073, -61.0498)
  line L10365 (203.073, -61.0498) -> (202.908, -61.1334)
  line L10366 (132.582, -59.6819) -> (132.669, -59.8456)
  line L10367 (202.755, -59.3171) -> (202.932, -59.3719)
  line L10368 (132.567, -60.7552) -> (132.445, -60.8956)
  line L10369 (124.788, -59.2626) -> (124.817, -58.9816)
  line L10370 (202.908, -61.1334) -> (202.729, -61.1832)
  line L10371 (159.605, -58.9458) -> (159.773, -58.987)
  line L10372 (132.158, -59.3318) -> (132.321, -59.42)
  line L10373 (203.491, -60.4581) -> (203.432, -60.6341)
  line L10374 (202.022, -61.0278) -> (201.881, -60.9076)
  line L10375 (132.299, -61.0097) -> (132.134, -61.0933)
  line L10376 (131.126, -59.5289) -> (131.27, -59.4127)
  line L10377 (130.907, -60.5573) -> (130.856, -60.3791)
  line L10378 (132.717, -60.4181) -> (132.658, -60.594)
  line L10379 (130.856, -60.3791) -> (130.84, -60.1943)
  line L10380 (201.691, -59.8734) -> (201.78, -59.7109)
  line L10381 (203.496, -60.0631) -> (203.514, -60.2477)
  line L10382 (126.976, -61.3166) -> (126.693, -61.3232)
  line L10383 (203.514, -60.2742) -> (203.491, -60.4581)
  line L10384 (201.681, -60.5974) -> (201.63, -60.4192)
  line L10385 (127.524, -61.185) -> (127.254, -61.2702)
  line L10386 (202.36, -61.1755) -> (202.184, -61.1182)
  line L10387 (202.184, -61.1182) -> (202.022, -61.0278)
  line L10388 (203.341, -60.7953) -> (203.219, -60.9356)
  line L10389 (202.386, -59.3145) -> (202.571, -59.2977)
  line L10390 (132.321, -59.42) -> (132.464, -59.5382)
  line L10391 (124.94, -60.0908) -> (124.85, -59.8228)
  line L10392 (125.418, -60.7834) -> (125.227, -60.576)
  line L10393 (127.254, -61.2702) -> (126.976, -61.3166)
  line L10394 (202.544, -61.1975) -> (202.36, -61.1755)
  line L10395 (131.981, -59.277) -> (132.158, -59.3318)
  line L10396 (203.514, -60.2477) -> (203.514, -60.2742)
  line L10397 (201.635, -60.0502) -> (201.691, -59.8734)
  line L10398 (201.881, -60.9076) -> (201.766, -60.7623)
  line L10399 (131.77, -61.1574) -> (131.586, -61.1354)
  line L10400 (130.917, -59.8334) -> (131.006, -59.6709)
  line L10401 (131.006, -59.6709) -> (131.126, -59.5289)
  line L10402 (201.766, -60.7623) -> (201.681, -60.5974)
  line L10403 (201.63, -60.4192) -> (201.614, -60.2344)
  line L10404 (132.74, -60.2076) -> (132.74, -60.2341)
  line L10405 (202.729, -61.1832) -> (202.544, -61.1975)
  line L10406 (125.133, -58.2013) -> (125.308, -57.9794)
  line L10407 (201.614, -60.2344) -> (201.635, -60.0502)
  line L10408 (158.251, -60.393) -> (158.096, -60.314)
  line L10409 (131.41, -61.0781) -> (131.248, -60.9877)
  line L10410 (157.824, -59.3909) -> (157.911, -59.2407)
  line L10411 (176.013, -58.987) -> (176.168, -59.066)
  line L10412 (176.353, -60.1393) -> (176.233, -60.2654)
  line L10413 (174.659, -60.4342) -> (174.491, -60.393)
  line L10414 (159.773, -58.987) -> (159.928, -59.066)
  line L10415 (174.752, -58.94) -> (175.752, -58.94)
  line L10416 (175.752, -58.94) -> (175.845, -58.9458)
  line L10417 (-1.0366, -57.9522) -> (-0.8594, -58.007)
  line L10418 (132.74, -60.2341) -> (132.717, -60.4181)
  line L10419 (-0.5535, -58.2134) -> (-0.4363, -58.3571)
  line L10420 (-0.8594, -58.007) -> (-0.6964, -58.0952)
  line L10421 (-0.2957, -58.6983) -> (-0.2776, -58.8828)
  line L10422 (174.003, -59.7306) -> (174.014, -59.5572)
  line L10423 (174.336, -60.314) -> (174.203, -60.2015)
  line L10424 (174.033, -59.9018) -> (174.003, -59.7306)
  line L10425 (158.176, -59.0194) -> (158.339, -58.9601)
  line L10426 (160.231, -59.4782) -> (160.261, -59.6494)
  line L10427 (159.993, -60.2654) -> (159.848, -60.3606)
  line L10428 (-0.6964, -58.0952) -> (-0.5535, -58.2134)
  line L10429 (176.49, -59.8228) -> (176.44, -59.9891)
  line L10430 (175.925, -60.4199) -> (175.752, -60.44)
  line L10431 (131.248, -60.9877) -> (131.107, -60.8675)
  line L10432 (157.774, -59.5572) -> (157.824, -59.3909)
  line L10433 (176.088, -60.3606) -> (175.925, -60.4199)
  line L10434 (160.163, -59.3184) -> (160.231, -59.4782)
  line L10435 (-0.4363, -58.3571) -> (-0.3493, -58.5208)
  line L10436 (176.44, -59.9891) -> (176.353, -60.1393)
  line L10437 (160.2, -59.9891) -> (160.113, -60.1393)
  line L10438 (160.25, -59.8228) -> (160.2, -59.9891)
  line L10439 (158.339, -58.9601) -> (158.512, -58.94)
  line L10440 (175.845, -58.9458) -> (176.013, -58.987)
  line L10441 (158.512, -60.44) -> (158.419, -60.4342)
  line L10442 (159.512, -60.44) -> (158.512, -60.44)
  line L10443 (157.763, -59.7306) -> (157.774, -59.5572)
  line L10444 (159.928, -59.066) -> (160.061, -59.1785)
  line L10445 (160.261, -59.6494) -> (160.25, -59.8228)
  line L10446 (158.031, -59.1146) -> (158.176, -59.0194)
  line L10447 (131.434, -59.3268) -> (131.612, -59.2744)
  line L10448 (176.301, -59.1785) -> (176.403, -59.3184)
  line L10449 (176.403, -59.3184) -> (176.471, -59.4782)
  line L10450 (130.992, -60.7222) -> (130.907, -60.5573)
  line L10451 (174.014, -59.5572) -> (174.064, -59.3909)
  line L10452 (174.416, -59.0194) -> (174.579, -58.9601)
  line L10453 (160.113, -60.1393) -> (159.993, -60.2654)
  line L10454 (-0.3493, -58.5208) -> (-0.2957, -58.6983)
  line L10455 (174.203, -60.2015) -> (174.101, -60.0616)
  line L10456 (158.096, -60.314) -> (157.963, -60.2015)
  line L10457 (176.233, -60.2654) -> (176.088, -60.3606)
  line L10458 (157.861, -60.0616) -> (157.793, -59.9018)
  line L10459 (158.419, -60.4342) -> (158.251, -60.393)
  line L10460 (157.793, -59.9018) -> (157.763, -59.7306)
  line L10461 (159.848, -60.3606) -> (159.685, -60.4199)
  line L10462 (158.512, -58.94) -> (159.512, -58.94)
  line L10463 (157.963, -60.2015) -> (157.861, -60.0616)
  line L10464 (157.911, -59.2407) -> (158.031, -59.1146)
  line L10465 (160.061, -59.1785) -> (160.163, -59.3184)
  line L10466 (159.685, -60.4199) -> (159.512, -60.44)
  line L10467 (159.512, -58.94) -> (159.605, -58.9458)
  line L10468 (176.168, -59.066) -> (176.301, -59.1785)
  line L10469 (132.658, -60.594) -> (132.567, -60.7552)
  line L10470 (131.107, -60.8675) -> (130.992, -60.7222)
  line L10471 (132.445, -60.8956) -> (132.299, -61.0097)
  line L10472 (-1.2475, -59.8326) -> (-1.4316, -59.8106)
  line L10473 (-2.1568, -58.6853) -> (-2.1008, -58.5085)
  line L10474 (122.153, -57.5676) -> (122.316, -57.6557)
  line L10475 (122.316, -57.6557) -> (122.459, -57.7739)
  line L10476 (-0.278, -58.9093) -> (-0.3012, -59.0932)
  line L10477 (174.151, -59.2407) -> (174.271, -59.1146)
  line L10478 (-0.5724, -59.5707) -> (-0.7186, -59.6849)
  line L10479 (122.716, -58.2588) -> (122.735, -58.4433)
  line L10480 (122.734, -58.4699) -> (122.711, -58.6538)
  line L10481 (120.901, -58.7931) -> (120.85, -58.6148)
  line L10482 (-1.7698, -59.6629) -> (-1.911, -59.5427)
  line L10483 (-2.0114, -58.3461) -> (-1.8923, -58.204)
  line L10484 (120.85, -58.6148) -> (120.835, -58.4301)
  line L10485 (176.501, -59.6494) -> (176.49, -59.8228)
  line L10486 (-1.4056, -57.9496) -> (-1.221, -57.9328)
  line L10487 (-2.1008, -58.5085) -> (-2.0114, -58.3461)
  line L10488 (120.835, -58.4301) -> (120.855, -58.2458)
  line L10489 (-0.3012, -59.0932) -> (-0.3597, -59.2692)
  line L10490 (121.101, -59.1033) -> (120.986, -58.958)
  line L10491 (-0.884, -59.7685) -> (-1.0626, -59.8183)
  line L10492 (121.001, -57.9066) -> (121.12, -57.7646)
  line L10493 (121.12, -57.7646) -> (121.264, -57.6484)
  line L10494 (174.064, -59.3909) -> (174.151, -59.2407)
  line L10495 (-0.7186, -59.6849) -> (-0.884, -59.7685)
  line L10496 (174.101, -60.0616) -> (174.033, -59.9018)
  line L10497 (122.663, -58.0813) -> (122.716, -58.2588)
  line L10498 (122.561, -58.9909) -> (122.44, -59.1313)
  line L10499 (122.735, -58.4433) -> (122.734, -58.4699)
  line L10500 (120.855, -58.2458) -> (120.911, -58.0691)
  line L10501 (-2.1109, -59.2325) -> (-2.162, -59.0543)
  line L10502 (122.294, -59.2454) -> (122.128, -59.329)
  line L10503 (121.765, -59.3931) -> (121.581, -59.3712)
  line L10504 (121.429, -57.5625) -> (121.607, -57.5102)
  line L10505 (122.576, -57.9176) -> (122.663, -58.0813)
  line L10506 (122.128, -59.329) -> (121.95, -59.3789)
  line L10507 (122.711, -58.6538) -> (122.652, -58.8297)
  line L10508 (-1.0626, -59.8183) -> (-1.2475, -59.8326)
  line L10509 (176.471, -59.4782) -> (176.501, -59.6494)
  line L10510 (122.652, -58.8297) -> (122.561, -58.9909)
  line L10511 (175.752, -60.44) -> (174.752, -60.44)
  line L10512 (-1.911, -59.5427) -> (-2.0261, -59.3974)
  line L10513 (-0.3597, -59.2692) -> (-0.4513, -59.4304)
  line L10514 (-1.221, -57.9328) -> (-1.0366, -57.9522)
  line L10515 (174.752, -60.44) -> (174.659, -60.4342)
  line L10516 (-2.0261, -59.3974) -> (-2.1109, -59.2325)
  line L10517 (121.976, -57.5127) -> (122.153, -57.5676)
  line L10518 (-1.6079, -59.7533) -> (-1.7698, -59.6629)
  line L10519 (174.579, -58.9601) -> (174.752, -58.94)
  line L10520 (-1.5835, -58.002) -> (-1.4056, -57.9496)
  line L10521 (121.95, -59.3789) -> (121.765, -59.3931)
  line L10522 (212.577, -57.5334) -> (212.761, -57.5528)
  line L10523 (121.404, -59.3139) -> (121.242, -59.2234)
  line L10524 (174.491, -60.393) -> (174.336, -60.314)
  line L10525 (-2.1775, -58.8695) -> (-2.1568, -58.6853)
  line L10526 (-0.2776, -58.8828) -> (-0.278, -58.9093)
  line L10527 (121.581, -59.3712) -> (121.404, -59.3139)
  line L10528 (120.986, -58.958) -> (120.901, -58.7931)
  line L10529 (122.459, -57.7739) -> (122.576, -57.9176)
  line L10530 (-1.7478, -58.0878) -> (-1.5835, -58.002)
  line L10531 (-2.162, -59.0543) -> (-2.1775, -58.8695)
  line L10532 (174.271, -59.1146) -> (174.416, -59.0194)
  line L10533 (-1.4316, -59.8106) -> (-1.6079, -59.7533)
  line L10534 (-1.8923, -58.204) -> (-1.7478, -58.0878)
  line L10535 (-0.4513, -59.4304) -> (-0.5724, -59.5707)
  line L10536 (38.4966, -57.8632) -> (38.3766, -57.6231)
  line L10537 (38.2603, -56.5693) -> (38.325, -56.3089)
  line L10538 (38.5605, -55.828) -> (38.7267, -55.6173)
  line L10539 (40.0425, -58.7939) -> (39.776, -58.7623)
  line L10540 (39.8939, -55.011) -> (40.1618, -54.9962)
  line L10541 (39.3774, -55.1523) -> (39.6306, -55.0633)
  line L10542 (38.2917, -57.3685) -> (38.2435, -57.1045)
  line L10543 (40.5755, -58.7435) -> (40.3108, -58.7876)
  line L10544 (38.325, -56.3089) -> (38.4257, -56.0601)
  line L10545 (39.776, -58.7623) -> (39.5166, -58.6936)
  line L10546 (41.2965, -58.3973) -> (41.0734, -58.5464)
  line L10547 (294.941, -54.9228) -> (295.175, -55.054)
  line L10548 (295.736, -55.6239) -> (295.864, -55.8601)
  line L10549 (296.028, -56.7613) -> (295.993, -57.0273)
  line L10550 (40.8314, -58.6626) -> (40.5755, -58.7435)
  line L10551 (38.3766, -57.6231) -> (38.2917, -57.3685)
  line L10552 (38.4257, -56.0601) -> (38.5605, -55.828)
  line L10553 (121.242, -59.2234) -> (121.101, -59.1033)
  line L10554 (39.5166, -58.6936) -> (39.2694, -58.5889)
  line L10555 (39.0395, -58.4505) -> (38.8314, -58.281)
  line L10556 (41.9566, -56.3659) -> (42.013, -56.6283)
  line L10557 (41.6691, -58.0128) -> (41.4964, -58.2182)
  line L10558 (121.607, -57.5102) -> (121.791, -57.4934)
  line L10559 (41.8637, -56.1141) -> (41.9566, -56.3659)
  line L10560 (39.2694, -58.5889) -> (39.0395, -58.4505)
  line L10561 (121.791, -57.4934) -> (121.976, -57.5127)
  line L10562 (42.013, -56.6283) -> (42.032, -56.896)
  line L10563 (294.429, -54.7654) -> (294.691, -54.826)
  line L10564 (295.864, -55.8601) -> (295.957, -56.1119)
  line L10565 (296.032, -56.642) -> (296.028, -56.7613)
  line L10566 (39.1393, -55.276) -> (39.3774, -55.1523)
  line L10567 (42.032, -56.896) -> (42.0283, -57.0153)
  line L10568 (41.8112, -57.7851) -> (41.6691, -58.0128)
  line L10569 (38.6492, -58.084) -> (38.4966, -57.8632)
  line L10570 (38.8314, -58.281) -> (38.6492, -58.084)
  line L10571 (294.691, -54.826) -> (294.941, -54.9228)
  line L10572 (295.388, -55.2168) -> (295.577, -55.408)
  line L10573 (38.9209, -55.432) -> (39.1393, -55.276)
  line L10574 (40.6907, -55.08) -> (40.941, -55.1768)
  line L10575 (295.993, -57.0273) -> (295.92, -57.2856)
  line L10576 (41.4964, -58.2182) -> (41.2965, -58.3973)
  line L10577 (40.941, -55.1768) -> (41.1751, -55.308)
  line L10578 (295.669, -57.7588) -> (295.496, -57.9642)
  line L10579 (41.0734, -58.5464) -> (40.8314, -58.6626)
  line L10580 (38.7267, -55.6173) -> (38.9209, -55.432)
  line L10581 (296.013, -56.3743) -> (296.032, -56.642)
  line L10582 (40.1618, -54.9962) -> (40.4292, -55.0194)
  line L10583 (41.5768, -55.662) -> (41.7362, -55.8779)
  line L10584 (40.3108, -58.7876) -> (40.0425, -58.7939)
  line L10585 (40.4292, -55.0194) -> (40.6907, -55.08)
  line L10586 (41.9197, -57.5396) -> (41.8112, -57.7851)
  line L10587 (295.957, -56.1119) -> (296.013, -56.3743)
  line L10588 (121.264, -57.6484) -> (121.429, -57.5625)
  line L10589 (41.1751, -55.308) -> (41.3885, -55.4708)
  line L10590 (41.9925, -57.2813) -> (41.9197, -57.5396)
  line L10591 (295.92, -57.2856) -> (295.811, -57.5311)
  line L10592 (122.44, -59.1313) -> (122.294, -59.2454)